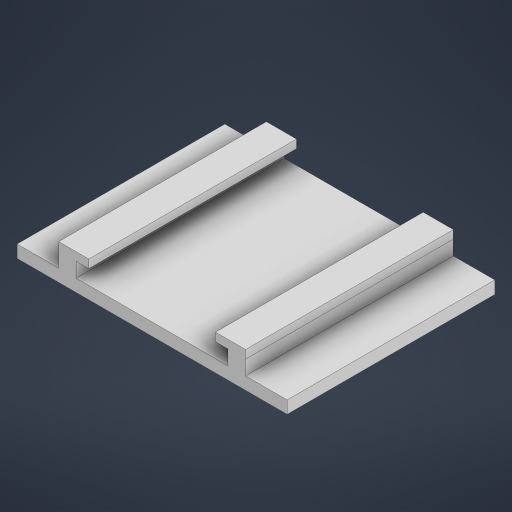
# Autodesk Inventor part: DINsupport
Saved by Autodesk Inventor 2023 (Build 270158000, 158)
## iProperties
Created: 2022-09-20
Part Number: DINsupport
Material: Generic
Document SubType Name: Modeling
Designer: CB110-09
Density: 1 g/cm^3
Appearance: Default
Author: CB110-09
Autodesk Inventor part; units mm, degrees
ref_plane "YZ Plane" through (0, 0, 0) normal (1, 0, 0) x (0, 1, 0)
ref_plane "XZ Plane" through (0, 0, 0) normal (0, 1, 0) x (-1, 0, 0)
ref_plane "XY Plane" through (0, 0, 0) normal (0, 0, 1) x (1, 0, 0)
sketch "Sketch1" plane through (0, 0, 0) normal (0, 1, 0) x (-1, 0, 0)
  line L0 (-32.5, 25) -> (32.5, 25)
  line L1 (32.5, 25) -> (32.5, -25)
  line L2 (32.5, -25) -> (-32.5, -25)
  line L3 (-32.5, -25) -> (-32.5, 25)
  line L4 (-32.5, 25) -> (32.5, -25) construction
  line L5 (32.5, 25) -> (-32.5, -25) construction
  point P0 (0, 0)
  dimension "d0" = 65
  dimension "d1" = 50
  constraints: 12 end point, 2 midpoint, 2 parallel, 1 horizontal, 1 perpendicular
  measures "d0" distance of L1.end L2.end
  measures "d1" distance of L0.end L1.end
extrude "Extrusion1" add sketch "Sketch1" along normal blind 3
sketch "Sketch2" plane through (0, 3, 0) normal (0, 1, 0) x (1, 0, 0)
  line L0 (32.5, 25) -> (-32.5, 25) projected
  line L1 (-18.25, -25) -> (18.25, -25)
  line L2 (18.25, -25) -> (18.25, 25)
  line L3 (18.25, 25) -> (-18.25, 25)
  line L4 (-18.25, 25) -> (-18.25, -25)
  line L5 (-18.25, -25) -> (18.25, 25) construction
  line L6 (18.25, -25) -> (-18.25, 25) construction
  line L7 (-22.5, -25) -> (22.5, -25)
  line L8 (22.5, -25) -> (22.5, 25)
  line L9 (22.5, 25) -> (-22.5, 25)
  line L10 (-22.5, 25) -> (-22.5, -25)
  line L11 (-22.5, -25) -> (22.5, 25) construction
  line L12 (22.5, -25) -> (-22.5, 25) construction
  point P0 (0, 0)
  dimension "d4" = 36.5
  dimension "d5" = 45
  constraints: 24 end point, 4 midpoint, 4 parallel, 2 horizontal, 2 perpendicular, 2 point on line
  measures "d4" distance of L3.end L2.end
  measures "d5" distance of L9.end L8.end
extrude "Extrusion2" add sketch "Sketch2" along normal blind 3.5 contours L8 L7 L2 L0 | L4 L7 L10 L0
sketch "Sketch3" plane through (0, 6.5, 0) normal (0, 1, 0) x (1, 0, 0)
  line L0 (-22.5, 25) -> (-32.5, 25) projected
  line L1 (-22.5, 25) -> (-15.25, 25)
  line L2 (-15.25, 25) -> (-15.25, -25)
  line L3 (-15.25, -25) -> (-22.5, -25)
  line L4 (-22.5, -25) -> (-22.5, 25)
  line L5 (-32.5, -25) -> (32.5, -25) projected
  line L6 (32.5, 25) -> (-32.5, 25) projected
  line L7 (22.4999, -25) -> (15.2499, -25)
  line L8 (15.2499, -25) -> (15.2499, 25)
  line L9 (15.2499, 25) -> (22.4999, 25)
  line L10 (22.4999, 25) -> (22.4999, -25)
  point P0 (0, 0)
  dimension "d8" = 7.25
  dimension "d9" = 7.25
  constraints: 16 end point, 4 parallel, 2 horizontal, 2 perpendicular, 2 point on line
  measures "d8" distance of L2.end L3.end
  measures "d9" distance of L8.end L9.end
extrude "Extrusion3" add sketch "Sketch3" along normal blind 2 contours L1 L2 L3 L4 | L6 L10 L5 L8
body "Solid1"
